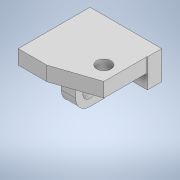
# Autodesk Inventor part: 件30
Saved by Autodesk Inventor 2020 (Build 240168000, 168)
## iProperties
Created: 2020-10-30
Part Number: 件30
Material: 一般
Document SubType Name: Modeling
Designer: USER
Density: 1 g/cm^3
Appearance: 預設
Author: USER
Autodesk Inventor part; units mm, degrees
ref_plane "YZ Plane" through (0, 0, 0) normal (1, 0, 0) x (0, 1, 0)
ref_plane "XZ Plane" through (0, 0, 0) normal (0, 1, 0) x (-1, 0, 0)
ref_plane "XY Plane" through (0, 0, 0) normal (0, 0, 1) x (1, 0, 0)
sketch "草圖1" plane through (0, 0, 0) normal (0, 0, 1) x (1, 0, 0)
  line L0 (25, -10) -> (-25, -10)
  line L1 (-25, -10) -> (-25, 10)
  line L2 (-25, 10) -> (25, 10)
  line L3 (25, 10) -> (25, -10)
  line L4 (25, -10) -> (-25, 10) construction
  line L5 (-25, -10) -> (25, 10) construction
  point P0 (0, 0)
  dimension "d0" = 50
  dimension "d1" = 20
  constraints: 12 end point, 2 midpoint, 2 parallel, 1 horizontal, 1 perpendicular
  measures "d0" distance between parallel lines of L3 L1
  measures "d1" distance between parallel lines of L0 L2
extrude "擠出1" add sketch "草圖1" along normal blind 10
sketch "草圖2" plane through (-25, -10, 0) normal (0, -1, 0) x (1, 0, 0)
  line L0 (0, 10) -> (0, 20)
  line L1 (0, 20) -> (10, 20)
  line L2 (50, 0) -> (50, 10) projected
  line L3 (0, 10) -> (50, 10) projected
  line L4 (10, 20) -> (40, 10)
  point P0 (25, 0)
  dimension "d4" = 10
  dimension "d5" = 10
  dimension "d6" = 40
  constraints: 6 end point, 1 perpendicular, 1 point on line, 1 vertical
  measures "d4" distance between parallel lines of L3 L1
  measures "d5" distance of L1.end L0.end
  measures "d6" distance of L4.end L0.start
extrude "擠出2" add sketch "草圖2" against normal blind 10
sketch "草圖3" plane through (-25, -10, 0) normal (0, -1, 0) x (1, 0, 0)
  line L0 (0, 0) -> (0, 20) projected
  line L1 (0, 0) -> (50, 0) projected
  line L2 (0, 20) -> (10, 20)
  line L3 (10, 20) -> (10, 0)
  line L4 (10, 0) -> (0, 0)
  line L5 (0, 0) -> (0, 20)
  point P0 (25, 0)
  dimension "d9" = 10
  constraints: 8 end point, 2 parallel, 1 horizontal, 1 perpendicular, 1 point on line
  measures "d9" distance between parallel lines of L0 L3
extrude "擠出3" add sketch "草圖3" along normal blind 30
fillet "圓角1" radius 10 1 edges at (-20, -40, 20)
sketch "草圖4" plane through (-15, -10, 20) normal (1, 0, 0) x (0, 0, -1)
  circle A0 centre (10, -20) radius 5
  line L0 (20, 0) -> (20, -30) projected
  line L1 (20, -30) -> (10, -30) projected
  point P0 (20, 10)
  dimension "d13" = 10
  dimension "d14" = 10
  dimension "d15" = 10
  constraints: 1 centre point
  measures "d13" distance from line of L0 A0.centre
  measures "d14" distance from line of L1 A0.centre
  measures "d15" diameter of A0
extrude "擠出4" cut sketch "草圖4" against normal blind 30
sketch "草圖5" plane through (-25, 0, 0) normal (0, 1, 0) x (1, 0, 0)
  line L0 (0, -20) -> (0, -10) projected
  line L1 (0, -10) -> (0, -50)
  line L2 (49.7047, -10) -> (49.7047, -40)
  line L3 (49.7047, -40) -> (20, -50)
  line L4 (20, -50) -> (0, -50)
  line L5 (50, -10) -> (0, -10) projected
  circle A0 centre (39.7047, -30) radius 5
  point P0 (25, 0)
  dimension "d18" = 40
  dimension "d19" = 30
  dimension "d20" = 20
  dimension "d21" = 10
  dimension "d22" = 20
  dimension "d23" = 10
  constraints: 8 end point, 2 vertical, 1 centre point, 1 horizontal, 1 horizontal alignment
  measures "d18" distance between parallel lines of L5 L4
  measures "d19" distance from line of L5 L2.end
  measures "d20" distance from line of L1 L3.end
  measures "d21" distance from line of L2 A0.centre
  measures "d22" distance from line of L4 A0.centre
  measures "d23" diameter of A0
extrude "擠出5" add sketch "草圖5" along normal blind 10
